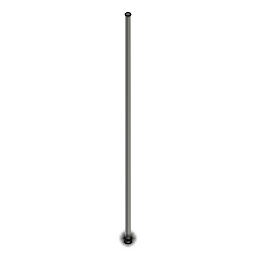
montare_finala (Autodesk Fusion 360 archive; units mm, degrees)
design "bara_vert"
part number: 2026-05-30-21-56-48-010
part number: 2026-05-30-21-58-53-842
Autodesk Fusion 360 part; units mm, degrees
sketch "Bara_vert" plane through (0, 0, 0) normal (0, 0, 1) x (1, 0, 0)
  circle A0 centre (0, 0) radius 2.25
  dimension "d1" = 4.5
  constraint coincident A0.centre origin
  measures "d1" diameter of A0
extrude "Extrude1" add sketch "Bara_vert" along normal blind 210 makes body 1
copy_body "Body->Comp1" bodies 1 removing the originals makes body 2 in component "Bara_vert"
move_face "MoveFace1" to x (1, 0, 0) y (0, 1, 0) z (0, 0, 1) at (0, 30, 0) 1 faces at (-0.877, -2.072, 140) on bodies 2 in component "Bara_vert"
sketch "Sketch1" plane through (0, 0, 0) normal (0, 0, -1) x (1, 0, 0) in component "Bara_vert"
  circle A0 centre (0, -30) radius 2.25
  circle A1 centre (0, -30) radius 2.75
  dimension "d4" = 5.5
  constraint concentric A0 A1
  measures "d4" diameter of A1
extrude "Extrude2" add sketch "Sketch1" along normal blind 3 contours A0 | A1 bodies 2 in component "Bara_vert"
component "Bara_vert" placed x (1, 0, 0) y (0, 1, 0) z (0, 0, 1) at (0, 0, 0)

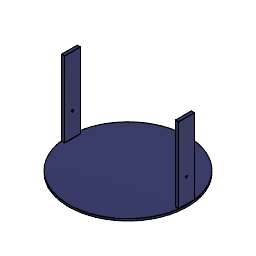
design "baza+laterale"
part number: 2026-05-30-21-15-33-105
part number: 2026-05-30-21-35-46-726
Autodesk Fusion 360 part; units mm, degrees
sketch "Baza" plane through (0, 0, 0) normal (0, 0, 1) x (1, 0, 0)
  circle A0 centre (0, 0) radius 150
  line L0 (0, 0) -> (0, 150) construction
  line L1 (0, 0) -> (-140, 0) construction
  line L2 (-140, 0) -> (-140, -20)
  line L3 (-140, 0) -> (-140, 20)
  line L4 (-140, 20) -> (-148, 20)
  line L5 (-148, 20) -> (-148, -20)
  line L6 (-148, -20) -> (-140, -20)
  line L7 (148, 20) -> (148, -20)
  line L8 (140, 0) -> (140, 20)
  line L9 (140, 0) -> (140, -20)
  line L10 (140, 20) -> (148, 20)
  line L11 (148, -20) -> (140, -20)
  dimension "d1" = 300
  dimension "d2" = 140
  dimension "d3" = 20
  dimension "d4" = 20
  dimension "d5" = 8
  constraint coincident A0.centre L0.start
  constraint coincident A0 L0.end
  constraint vertical L0
  constraint perpendicular L0 L1
  constraint perpendicular L1 L2
  constraint perpendicular L1 L3
  constraint perpendicular L3 L4
  constraint perpendicular L4 L5
  constraint perpendicular L2 L6
  constraint symmetric L0 L1.end L8.start
  constraint symmetric L0 L2.end L9.end
  constraint symmetric L0 L3.end L8.end
  constraint symmetric L0 L4.end L7.start
  constraint symmetric L0 L5.end L7.end
  measures "d1" diameter of A0
  measures "d2" distance of A0.centre L1.end
  measures "d3" distance of L1.end L2.end
  measures "d4" distance of L1.end L3.end
  measures "d5" distance of L3.end L4.end
extrude "Extrude1" add sketch "Baza" along normal blind 190 from surface at 5 contours L2 L3 L4 L5 L6 | L7 L8 L9 L10 L11 makes body 1 at (-140, 6.6667, 68.3333) makes body 2 at (148, 6.6667, 68.3333)
extrude "Extrude2" add sketch "Baza" along normal blind 5 contours A0 | L2 L3 L4 L5 L6 | L7 L8 L9 L10 L11 bodies 1 2
sketch "side_hole" plane through (-140, 0, 0) normal (1, 0, 0) x (0, 1, 0)
  line L0 (-20, 5) -> (20, 5)
  line L1 (20, 5) -> (20, 195)
  line L2 (20, 195) -> (-20, 195)
  line L3 (-20, 195) -> (-20, 5)
  line L4 (0, 5) -> (0, 65) construction
  circle A0 centre (0, 65) radius 2.5
  dimension "d12" = 60
  dimension "d13" = 5
  constraint midpoint L0 L4.start
  constraint perpendicular L0 L4
  constraint coincident L4.end A0.centre
  measures "d12" distance of L4.start L4.end
  measures "d13" diameter of A0
extrude "Extrude3" cut sketch "side_hole" along normal blind 600 and the other way blind 100 contours A0 bodies 1
copy_body "Body->Comp1" bodies 1 removing the originals makes body 3 in component "Baza+laterale"
component "Baza+laterale" placed x (1, 0, 0) y (0, 1, 0) z (0, 0, 1) at (0, 0, 0)

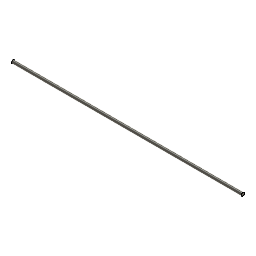
design "bara_32cm"
part number: 2026-05-30-21-52-07-364
part number: 2026-05-30-21-56-40-269
Autodesk Fusion 360 part; units mm, degrees
sketch "Bara_32cm" plane through (0, 0, 0) normal (1, 0, 0) x (0, 1, 0)
  circle A0 centre (0, 0) radius 2.25
  dimension "d1" = 4.5
  constraint coincident A0.centre origin
  measures "d1" diameter of A0
extrude "Extrude1" add sketch "Bara_32cm" along normal blind 320
component "bara_32cm (1)" placed x (1, 0, 0) y (0, 1, 0) z (0, 0, 1) at (0, 0, 0)
